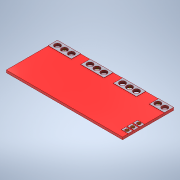
# Autodesk Inventor part: CARGADOR BATERIA LIPO LITIO 4 CELDAS 5A 18650
Saved by Autodesk Inventor 2020 (Build 240168000, 168)
## iProperties
Created: 2021-12-16
Part Number: CARGADOR BATERIA LIPO LITIO 4 CELDAS 5A 18650
Material: Genérico
Document SubType Name: Modeling
Designer: DANIEL
Density: 1 g/cm^3
Appearance: Rojo
Author: DANIEL
Autodesk Inventor part; units mm, degrees
ref_plane "YZ Plane" through (0, 0, 0) normal (1, 0, 0) x (0, 1, 0)
ref_plane "XZ Plane" through (0, 0, 0) normal (0, 1, 0) x (-1, 0, 0)
ref_plane "XY Plane" through (0, 0, 0) normal (0, 0, 1) x (1, 0, 0)
sketch "Boceto1" plane through (0, 0, 0) normal (0, 1, 0) x (-1, 0, 0)
  line L0 (25, 11) -> (-25, 11)
  line L1 (-25, 11) -> (-25, -11)
  line L2 (-25, -11) -> (25, -11)
  line L3 (25, -11) -> (25, 11)
  point P0 (0, 0)
  dimension "largo" = 50
  dimension "ancho" = 22
  dimension "d2" = 11
  dimension "d3" = 25
  constraints: 8 end point, 2 parallel, 1 horizontal, 1 perpendicular
  measures "largo" distance between parallel lines of L3 L1
  measures "ancho" distance between parallel lines of L2 L0
  measures "d2" distance from line of point (0, 0) L2
  measures "d3" distance from line of L3 point (0, 0)
extrude "Extrusión1" add sketch "Boceto1" along normal blind 1
sketch "Boceto2" plane through (0, 1, 0) normal (0, 1, 0) x (1, 0, 0)
  line L0 (-25, 11) -> (-25, -11) projected
  line L1 (-25, 7) -> (-15, 7)
  line L2 (-15, 7) -> (-15, 11)
  line L3 (-15, 11) -> (-25, 11)
  line L4 (-25, 11) -> (-25, 7)
  line L5 (-11, 11) -> (-1, 11)
  line L6 (-1, 11) -> (-1, 7)
  line L7 (-1, 7) -> (-11, 7)
  line L8 (-11, 7) -> (-11, 11)
  line L9 (25, 11) -> (-25, 11) projected
  line L10 (3, 11) -> (13, 11)
  line L11 (13, 11) -> (13, 7)
  line L12 (13, 7) -> (3, 7)
  line L13 (3, 7) -> (3, 11)
  line L14 (18.5, 11) -> (25, 11)
  line L15 (25, 11) -> (25, 7)
  line L16 (25, 7) -> (18.5, 7)
  line L17 (18.5, 7) -> (18.5, 11)
  line L18 (25, -11) -> (25, 11) projected
  line L19 (25, -3.5465) -> (22, -3.5465)
  line L20 (22, -3.5465) -> (22, -1.5465)
  line L21 (22, -1.5465) -> (25, -1.5465)
  line L22 (25, -1.5465) -> (25, -3.5465)
  line L23 (25, -4.0465) -> (22, -4.0465)
  line L24 (22, -4.0465) -> (22, -6.0465)
  line L25 (22, -6.0465) -> (25, -6.0465)
  line L26 (25, -6.0465) -> (25, -4.0465)
  line L27 (25, -6.5465) -> (22, -6.5465)
  line L28 (22, -6.5465) -> (22, -8.5465)
  line L29 (22, -8.5465) -> (25, -8.5465)
  line L30 (25, -8.5465) -> (25, -6.5465)
  point P0 (0, 0)
  point P1 (25, -1.5465)
  point P2 (25, 11)
  point P3 (13, 11)
  dimension "d6" = 10
  dimension "d7" = 4
  dimension "d8" = 10
  dimension "d9" = 4
  dimension "d10" = 10
  dimension "d11" = 4
  dimension "d12" = 6.5
  dimension "d13" = 4
  dimension "d14" = 3
  dimension "d15" = 2
  dimension "d22" = 0
  dimension "d23" = 0
  dimension "d24" = 14
  dimension "d25" = 14
  dimension "d27" = 0
  dimension "d28" = 2
  dimension "d29" = 3
  dimension "d30" = 2
  dimension "d31" = 0.5
  dimension "d32" = 0.5
  constraints: 56 end point, 14 parallel, 7 horizontal, 7 perpendicular, 6 point on line
  measures "d6" distance of L3.end L2.end
  measures "d7" distance of L2.end L1.end
  measures "d8" distance of L6.end L7.end
  measures "d9" distance of L5.end L6.end
  measures "d10" distance of L11.end L12.end
  measures "d11" distance of L10.end L11.end
  measures "d12" distance of L15.end L16.end
  measures "d13" distance of L14.end L15.end
  measures "d14" distance of L20.end L21.end
  measures "d15" distance of L19.end L20.end
  measures "d22" distance between parallel lines of L9 L3
  measures "d23" distance between parallel lines of L9 L5
  measures "d24" distance between parallel lines of L8 L0
  measures "d25" distance between parallel lines of L13 L8
  measures "d27" distance between parallel lines of L18 L15
  measures "d28" distance of L24.end L23.end
  measures "d29" distance of L29.end L28.end
  measures "d30" distance of L28.end L27.end
  measures "d31" distance between parallel lines of L19 L23
  measures "d32" distance between parallel lines of L27 L25
extrude "Extrusión2" add sketch "Boceto2" along normal blind 0.1
sketch "Boceto3" plane through (0, 1.1, 0) normal (0, 1, 0) x (1, 0, 0)
  circle A0 centre (-23, 9) radius 1.25
  circle A1 centre (-20, 9) radius 1.25
  circle A2 centre (-17, 9) radius 1.25
  line L0 (-15, 11) -> (-25, 11) projected
  line L1 (-25, 11) -> (-25, 7) projected
  line L2 (-25, 7) -> (-15, 7) projected
  circle A3 centre (-9, 9) radius 1.25
  circle A4 centre (-6, 9) radius 1.25
  circle A5 centre (-3, 9) radius 1.25
  line L3 (-11, 11) -> (-11, 7) projected
  circle A6 centre (5, 9) radius 1.25
  circle A7 centre (8, 9) radius 1.25
  circle A8 centre (11, 9) radius 1.25
  circle A9 centre (20.2, 9) radius 1.25
  circle A10 centre (23.2, 9) radius 1.25
  line L4 (18.5, 11) -> (18.5, 7) projected
  line L5 (3, 11) -> (3, 7) projected
  circle A11 centre (23.5, -7.5613) radius 0.75
  circle A12 centre (23.5, -5.1334) radius 0.75
  circle A13 centre (23.5, -2.4754) radius 0.75
  line L6 (22, -6.5465) -> (22, -8.5465) projected
  point P0 (0, 0)
  dimension "d33" = 2.5
  dimension "d34" = 2.5
  dimension "d35" = 2.5
  dimension "d36" = 2
  dimension "d37" = 2
  dimension "d38" = 3
  dimension "d39" = 2
  dimension "d40" = 3
  dimension "d41" = 2
  dimension "d42" = 2.5
  dimension "d43" = 2.5
  dimension "d44" = 2.5
  dimension "d45" = 3
  dimension "d46" = 3
  dimension "d47" = 2
  dimension "d48" = 2.5
  dimension "d49" = 2.5
  dimension "d50" = 2.5
  dimension "d51" = 3
  dimension "d52" = 3
  dimension "d53" = 2.5
  dimension "d54" = 2.5
  dimension "d56" = 3
  dimension "d58" = 1.7
  dimension "d59" = 2
  dimension "d60" = 1.5
  dimension "d61" = 1.5
  dimension "d62" = 1.5
  dimension "d63" = 1.5
  constraints: 14 centre point, 5 horizontal alignment, 2 vertical alignment
  measures "d33" diameter of A0
  measures "d34" diameter of A1
  measures "d35" diameter of A2
  measures "d36" distance from line of L0 A0.centre
  measures "d37" distance from line of L1 A0.centre
  measures "d38" distance of A0.centre A1.centre
  measures "d39" distance from line of L2 A1.centre
  measures "d40" distance of A1.centre A2.centre
  measures "d41" distance from line of L0 A2.centre
  measures "d42" diameter of A3
  measures "d43" diameter of A4
  measures "d44" diameter of A5
  measures "d45" distance of A3.centre A4.centre
  measures "d46" distance of A4.centre A5.centre
  measures "d47" distance from line of L3 A3.centre
  measures "d48" diameter of A6
  measures "d49" diameter of A7
  measures "d50" diameter of A8
  measures "d51" distance of A6.centre A7.centre
  measures "d52" distance of A7.centre A8.centre
  measures "d53" diameter of A9
  measures "d54" diameter of A10
  measures "d56" distance of A9.centre A10.centre
  measures "d58" distance from line of L4 A9.centre
  measures "d59" distance from line of L5 A6.centre
  measures "d60" diameter of A11
  measures "d61" diameter of A12
  measures "d62" diameter of A13
  measures "d63" distance from line of L6 A11.centre
extrude "Extrusión3" cut sketch "Boceto3" against normal blind 5.1
sketch "Boceto4" plane through (0, 1.1, 0) normal (0, 1, 0) x (1, 0, 0)
  circle A0 centre (-20, 9) radius 1.25 projected
sketch "Boceto5" plane through (0, 1.1, 0) normal (0, 1, 0) x (1, 0, 0)
  circle A0 centre (-6, 9) radius 1.25 projected
sketch "Boceto6" plane through (0, 1.1, 0) normal (0, 1, 0) x (1, 0, 0)
  circle A0 centre (8, 9) radius 1.25 projected
sketch "Boceto7" plane through (0, 1.1, 0) normal (0, 1, 0) x (1, 0, 0)
  circle A0 centre (20.2, 9) radius 1.25 projected
sketch "Boceto8" plane through (0, 1.1, 0) normal (0, 1, 0) x (1, 0, 0)
  circle A0 centre (23.5, -2.4754) radius 0.75 projected
sketch "Boceto9" plane through (0, 1.1, 0) normal (0, 1, 0) x (1, 0, 0)
  circle A0 centre (23.5, -5.1334) radius 0.75 projected
sketch "Boceto10" plane through (0, 1.1, 0) normal (0, 1, 0) x (1, 0, 0)
  circle A0 centre (23.5, -7.5613) radius 0.75 projected
equation "\"d2\" = 0.5 * ancho"
equation "\"d3\" = 0.5 * largo"
